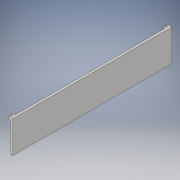
# Autodesk Inventor part: FrameTestinsidePlate
Saved by Autodesk Inventor 2017 (Build 210142000, 142)
## iProperties
Created: 2018-04-18
Part Number: FrameTestinsidePlate
Material: Generic
Document SubType Name: Modeling
Designer: User
Density: 1 g/cm^3
Appearance: Default
Author: User
Autodesk Inventor part; units mm, degrees
ref_plane "YZ Plane" through (0, 0, 0) normal (1, 0, 0) x (0, 1, 0)
ref_plane "XZ Plane" through (0, 0, 0) normal (0, 1, 0) x (-1, 0, 0)
ref_plane "XY Plane" through (0, 0, 0) normal (0, 0, 1) x (1, 0, 0)
sketch "Sketch1" plane through (0, 0, 0) normal (1, 0, 0) x (0, 1, 0)
  line L0 (-44.45, 222.25) -> (44.45, 222.25)
  line L1 (44.45, 222.25) -> (44.45, -222.25)
  line L2 (44.45, -222.25) -> (-44.45, -222.25)
  line L3 (-44.45, -222.25) -> (-44.45, 222.25)
  line L4 (-44.45, 222.25) -> (44.45, -222.25) construction
  line L5 (44.45, 222.25) -> (-44.45, -222.25) construction
  point P0 (0, 0)
  dimension "d0" = 88.9
  dimension "d1" = 444.5
  constraints: 12 end point, 2 midpoint, 2 parallel, 1 horizontal, 1 perpendicular
  measures "d0" distance of L1.end L2.end
  measures "d1" distance of L0.end L1.end
extrude "Extrusion1" add sketch "Sketch1" along normal blind 6.35
sketch "Sketch2" plane through (0, 0, 0) normal (-1, 0, 0) x (0, 0, 1)
  line L0 (-222.25, -44.45) -> (-222.25, 44.45) projected
  line L1 (-222.25, 44.45) -> (-209.55, 44.45)
  line L2 (-209.55, 44.45) -> (-209.55, 38.1)
  line L3 (-209.55, 38.1) -> (-222.25, 38.1)
  line L4 (-222.25, 38.1) -> (-222.25, 44.45)
  line L5 (-222.25, 44.45) -> (222.25, 44.45) projected
  line L6 (222.25, 44.45) -> (209.55, 44.45)
  line L7 (209.55, 44.45) -> (209.55, 38.1)
  line L8 (209.55, 38.1) -> (222.25, 38.1)
  line L9 (222.25, 38.1) -> (222.25, 44.45)
  line L10 (222.25, -44.45) -> (-222.25, -44.45) projected
  line L11 (-101.6, -44.45) -> (-88.9, -44.45)
  line L12 (-88.9, -44.45) -> (-88.9, -38.1)
  line L13 (-88.9, -38.1) -> (-101.6, -38.1)
  line L14 (-101.6, -38.1) -> (-101.6, -44.45)
  line L15 (88.9, -44.45) -> (101.6, -44.45)
  line L16 (101.6, -44.45) -> (101.6, -38.1)
  line L17 (101.6, -38.1) -> (88.9, -38.1)
  line L18 (88.9, -38.1) -> (88.9, -44.45)
  point P0 (0, 0)
  dimension "d4" = 12.7
  dimension "d5" = 6.35
  dimension "d6" = 6.35
  dimension "d7" = 12.7
  dimension "d8" = 6.35
  dimension "d9" = 12.7
  dimension "d10" = 12.7
  dimension "d11" = 88.9
  dimension "d12" = 88.9
  constraints: 32 end point, 8 parallel, 4 horizontal, 4 perpendicular, 3 point on line
  measures "d4" distance of L2.end L3.end
  measures "d5" distance of L1.end L2.end
  measures "d6" distance of L6.end L7.end
  measures "d7" distance of L7.end L8.end
  measures "d8" distance of L11.end L12.end
  measures "d9" distance between parallel lines of L14 L12
  measures "d10" distance of L16.end L17.end
  measures "d11" distance from line of L18 point (0, 0)
  measures "d12" horizontal distance of point (0, 0) L12.end
extrude "Extrusion2" add sketch "Sketch2" along normal blind 6.35
sketch "Sketch3" plane through (6.35, 44.45, 222.25) normal (0, 1, 0) x (1, 0, 0)
  line L0 (-6.35, 120.65) -> (-6.35, 0) projected
  line L1 (0, 0) -> (-12.7, 0) projected
  line L2 (-12.7, 431.8) -> (-12.7, 444.5) projected
  line L3 (0, 444.5) -> (-12.7, 444.5) projected
  line L4 (-6.35, 431.8) -> (-12.7, 431.8) projected
  line L5 (-6.35, 12.7) -> (-12.7, 12.7) projected
  line L6 (-12.7, 0) -> (-12.7, 12.7) projected
  point P0 (-6.35, 222.25)
  point P1 (-9.525, 6.35)
  point P2 (-9.525, 438.15)
  dimension "d44" = 3.175
  dimension "d45" = 6.35
  dimension "d46" = 6.35
  dimension "d47" = 3.175
  measures "d44" distance from line of L2 point (-9.525, 438.15)
  measures "d45" distance from line of L4 point (-9.525, 438.15)
  measures "d46" distance from line of L5 point (-9.525, 6.35)
  measures "d47" distance from line of L6 point (-9.525, 6.35)
sketch "Sketch4" plane through (6.35, -44.45, -222.25) normal (0, -1, 0) x (1, 0, 0)
  line L0 (-6.35, 311.15) -> (-6.35, 323.85)
  line L1 (-6.35, 431.8) -> (-6.35, 12.7)
  line L2 (-6.35, 120.65) -> (-12.7, 120.65) projected
  line L3 (-12.7, 120.65) -> (-12.7, 133.35) projected
  line L4 (-12.7, 311.15) -> (-12.7, 323.85) projected
  line L5 (-6.35, 323.85) -> (-12.7, 323.85) projected
  point P0 (-6.35, 222.25)
  point P1 (-9.525, 317.5)
  point P2 (-9.525, 127)
  dimension "d33" = 3.175
  dimension "d34" = 6.35
  dimension "d35" = 3.175
  dimension "d36" = 6.35
  constraints: 4 end point
  measures "d33" distance from line of L3 point (-9.525, 127)
  measures "d34" distance from line of point (-9.525, 127) L2
  measures "d35" distance from line of L4 point (-9.525, 317.5)
  measures "d36" distance from line of L5 point (-9.525, 317.5)
hole "Hole3" at (-3.175, -44.45, 95.25) at (-3.175, -44.45, -95.25) direction (0, 1, 0) diameter 5.08 depth 6.35 tip angle 118
hole "Hole4" at (-3.175, 44.45, 215.9) at (-3.175, 44.45, -215.9) direction (0, -1, 0) diameter 5.08 depth 6.35 tip angle 118
equation "\"d6\" = d5"
equation "\"d7\" = d4"
equation "\"d8\" = d5"
equation "\"d9\" = d4"
equation "\"d10\" = d9"
equation "\"d46\" = d45"
equation "\"d47\" = d44"
equation "\"d35\" = d33"
equation "\"d36\" = d34"
equation "\"d42\" = d15"
equation "\"d53\" = d15"
equation "\"d15\" = d17"
equation "\"d17\" = d16"
equation "\"d16\" = 6.35"
body "Solid1"
